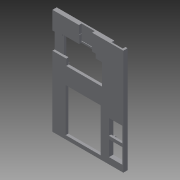
# Autodesk Inventor part: DisplayBottom2
Saved by Autodesk Inventor 2014 SP1 (Build 180222100, 222)
## iProperties
Created: 2014-03-24
Part Number: DisplayBottom2
Material: Generic
Document SubType Name: Modeling
Designer: patrigg
Density: 1 g/cm^3
Appearance: Default
Author: patrigg
Autodesk Inventor part; units mm, degrees
ref_plane "YZ Plane" through (0, 0, 0) normal (1, 0, 0) x (0, 1, 0)
ref_plane "XZ Plane" through (0, 0, 0) normal (0, 1, 0) x (-1, 0, 0)
ref_plane "XY Plane" through (0, 0, 0) normal (0, 0, 1) x (1, 0, 0)
sketch "Sketch2" plane through (0, 0, 0) normal (0, 1, 0) x (-1, 0, 0)
  line L0 (-33.5, -50) -> (33.5, -50)
  line L1 (33.5, -50) -> (33.5, 50)
  line L2 (33.5, 50) -> (-33.5, 50)
  line L3 (-33.5, 50) -> (-33.5, -50)
  line L4 (-33.5, -50) -> (33.5, 50) construction
  line L5 (33.5, -50) -> (-33.5, 50) construction
  point P0 (0, 0)
  dimension "d0" = 67
  dimension "d1" = 100
  constraints: 12 end point, 2 midpoint, 2 parallel, 1 horizontal, 1 perpendicular
  measures "d0" distance of L2.end L1.end
  measures "d1" distance of L1.end L0.end
extrude "Extrusion1" add sketch "Sketch2" along normal blind 4
sketch "Sketch3" plane through (0, 4, 0) normal (0, 1, 0) x (1, 0, 0)
  line L0 (33.5, 50) -> (-33.5, 50) projected
  line L1 (-23.5, -4.5) -> (14.5, -4.5)
  line L2 (14.5, -4.5) -> (14.5, 48)
  line L3 (14.5, 48) -> (-23.5, 48)
  line L4 (-23.5, 48) -> (-23.5, -4.5)
  line L5 (-23.5, -4.5) -> (14.5, 48) construction
  line L6 (14.5, -4.5) -> (-23.5, 48) construction
  line L7 (-33.5, 50) -> (-33.5, -50) projected
  point P0 (0, 0)
  point P1 (-4.5, 21.75)
  dimension "d4" = 38
  dimension "d5" = 52.5
  dimension "d6" = 2
  dimension "d111" = 10
  constraints: 12 end point, 2 midpoint, 2 parallel, 1 horizontal, 1 perpendicular
  measures "d4" distance of L3.end L2.end
  measures "d5" distance of L2.end L1.end
  measures "d6" distance between parallel lines of L0 L3
  measures "d111" distance between parallel lines of L4 L7
extrude "Extrusion2" cut sketch "Sketch3" against normal blind 1.5
sketch "Sketch4" plane through (0, 2.5, 0) normal (0, 1, 0) x (1, 0, 0)
  line L0 (14.5, -4.5) -> (-23.5, -4.5) projected
  line L1 (14.5, 48) -> (14.5, -4.5) projected
  line L2 (-23.5, 48) -> (14.5, 48) projected
  line L3 (-23.5, -4.5) -> (-23.5, 48) projected
  line L4 (-21, 46.5) -> (12, 46.5)
  line L5 (12, 46.5) -> (12, 5.5)
  line L6 (12, 5.5) -> (-21, 5.5)
  line L7 (-21, 5.5) -> (-21, 46.5)
  line L8 (-21, 46.5) -> (12, 5.5) construction
  line L9 (12, 46.5) -> (-21, 5.5) construction
  point P0 (0, 0)
  point P1 (-4.5, 26)
  dimension "d9" = 10
  dimension "d10" = 1.5
  dimension "d11" = 2.5
  dimension "d12" = 2.5
  constraints: 12 end point, 2 midpoint, 2 parallel, 1 horizontal, 1 perpendicular
  measures "d9" distance between parallel lines of L0 L6
  measures "d10" distance between parallel lines of L2 L4
  measures "d11" distance between parallel lines of L1 L5
  measures "d12" distance between parallel lines of L3 L7
extrude "Extrusion3" cut sketch "Sketch4" against normal blind 2.5 contours L4 L5 L6 L7
sketch "Sketch12" plane through (0, 4, 0) normal (0, 1, 0) x (1, 0, 0)
  line L0 (-24.5, -34.5) -> (13.5, -34.5)
  line L1 (13.5, -34.5) -> (13.5, -10.5)
  line L2 (13.5, -10.5) -> (-24.5, -10.5)
  line L3 (-24.5, -10.5) -> (-24.5, -34.5)
  line L4 (-24.5, -34.5) -> (13.5, -10.5) construction
  line L5 (13.5, -34.5) -> (-24.5, -10.5) construction
  line L6 (-23.5, -4.5) -> (-23.5, 48) projected
  line L7 (14.5, -4.5) -> (-23.5, -4.5) projected
  point P0 (0, 0)
  point P1 (-5.5, -22.5)
  point P2 (-5.5, -22.5)
  dimension "d58" = 38
  dimension "d59" = 24
  dimension "d112" = 1
  dimension "d154" = 6
  constraints: 12 end point, 3 midpoint, 2 parallel, 1 horizontal, 1 perpendicular
  measures "d58" distance of L2.end L1.end
  measures "d59" distance of L1.end L0.end
  measures "d112" distance between parallel lines of L3 L6
  measures "d154" distance between parallel lines of L7 L2
extrude "Extrusion10" cut sketch "Sketch12" against normal blind 4
sketch "Sketch18" plane through (13.5, 4, 10.5) normal (-1, 0, 0) x (0, 0, 1)
  line L0 (0, 0) -> (24, 0) projected
  line L1 (24, -4) -> (20, -4)
  line L2 (20, -4) -> (20, -1.8)
  line L3 (20, -1.8) -> (24, -1.8)
  line L4 (24, -1.8) -> (24, -4)
  point P0 (-10.5, -4)
  dimension "d88" = 4
  dimension "d89" = 1.8
  constraints: 8 end point, 2 parallel, 1 horizontal, 1 perpendicular
  measures "d88" distance of L2.end L3.end
  measures "d89" distance between parallel lines of L3 L0
extrude "Extrusion17" add sketch "Sketch18" along normal blind 6
sketch "Sketch20" plane through (-24.5, 4, 34.5) normal (1, 0, 0) x (0, 0, -1)
  line L0 (0, 0) -> (24, 0) projected
  line L1 (24, -4) -> (18, -4)
  line L2 (18, -4) -> (18, -1.8)
  line L3 (18, -1.8) -> (24, -1.8)
  line L4 (24, -1.8) -> (24, -4)
  point P0 (34.5, -4)
  dimension "d96" = 6
  dimension "d97" = 1.8
  constraints: 8 end point, 2 parallel, 1 horizontal, 1 perpendicular
  measures "d96" distance of L2.end L3.end
  measures "d97" distance between parallel lines of L3 L0
extrude "Extrusion19" add sketch "Sketch20" along normal blind 4
sketch "Sketch22" plane through (0, 0, 0) normal (0, -1, 0) x (1, 0, 0)
  line L0 (33.5, 50) -> (33.5, -50) projected
  line L1 (32.5, -44) -> (20, -44)
  line L2 (20, -44) -> (20, -12)
  line L3 (20, -12) -> (32.5, -12)
  line L4 (32.5, -12) -> (32.5, -44)
  line L5 (33.5, -50) -> (-33.5, -50) projected
  point P0 (0, 0)
  dimension "d102" = 1
  dimension "d103" = 12.5
  dimension "d110" = 32
  dimension "d155" = 6
  constraints: 8 end point, 2 parallel, 1 horizontal, 1 perpendicular
  measures "d102" distance between parallel lines of L4 L0
  measures "d103" distance between parallel lines of L2 L4
  measures "d110" distance between parallel lines of L3 L1
  measures "d155" distance between parallel lines of L5 L1
extrude "Extrusion21" cut sketch "Sketch22" against normal up to next
sketch "Sketch23" plane through (0, 4, 0) normal (0, 1, 0) x (1, 0, 0)
  line L0 (-24.5, -10.5) -> (13.5, -10.5) projected
  line L1 (14.5, 48) -> (14.5, -4.5) projected
  line L2 (14.5, -4.5) -> (-23.5, -4.5) projected
  line L3 (-23.5, -4.5) -> (-23.5, 48) projected
  line L4 (-21.5, -4.5) -> (-21.5, -10.5)
  line L5 (12.5, -4.5) -> (12.5, -10.5)
  point P0 (0, 0)
  dimension "d114" = 2
  dimension "d115" = 2
  constraints: 4 end point, 4 point on line, 2 perpendicular
  measures "d114" distance between parallel lines of L4 L3
  measures "d115" distance between parallel lines of L1 L5
extrude "Extrusion22" cut sketch "Sketch23" against normal up to surface (1.5 mm away)
sketch "Sketch24" plane through (32.5, 0, -44) normal (-1, 0, 0) x (0, 0, 1)
  line L0 (0, 0) -> (0, 4) projected
  line L1 (32, 0) -> (0, 0) projected
  line L2 (14.5, 0) -> (17.5, 0)
  line L3 (17.5, 0) -> (17.5, 2)
  line L4 (17.5, 2) -> (14.5, 2)
  line L5 (14.5, 2) -> (14.5, 0)
  line L6 (14.5, 0) -> (17.5, 2) construction
  line L7 (17.5, 0) -> (14.5, 2) construction
  point P0 (16, 1)
  dimension "d118" = 3
  dimension "d119" = 2
  dimension "d120" = 16
  constraints: 12 end point, 2 midpoint, 2 parallel, 1 collinear, 1 horizontal, 1 perpendicular
  measures "d118" distance of L4.end L3.end
  measures "d119" distance of L3.end L2.end
  measures "d120" distance from line of L0 point (16, 1)
extrude "Extrusion23" add sketch "Sketch24" along normal up to next
sketch "Sketch25" plane through (32.5, 2, -26.5) normal (0, 1, 0) x (1, 0, 0)
  line L0 (0, 0) -> (-12.5, 0) projected
  line L1 (0, 3) -> (-12.5, 3) projected
  line L2 (-7.75, 1) -> (-4.75, 1)
  line L3 (-4.75, 1) -> (-4.75, 3)
  line L4 (-4.75, 3) -> (-7.75, 3)
  line L5 (-7.75, 3) -> (-7.75, 1)
  line L6 (-7.75, 1) -> (-4.75, 3) construction
  line L7 (-4.75, 1) -> (-7.75, 3) construction
  point P0 (-32.5, -26.5)
  point P1 (-6.25, 2)
  point P2 (-6.25, 2)
  point P3 (-6.25, 0)
  dimension "d123" = 3
  dimension "d124" = 2
  constraints: 12 end point, 4 midpoint, 2 parallel, 1 collinear, 1 horizontal, 1 perpendicular, 1 vertical alignment
  measures "d123" distance of L4.end L3.end
  measures "d124" distance of L3.end L2.end
extrude "Extrusion24" cut sketch "Sketch25" against normal blind 0.5
fillet "Fillet6" radius 1 1 edges at (26.25, 1.5, -29.5)
sketch "Sketch26" plane through (32.5, 2, -26.5) normal (0, 1, 0) x (1, 0, 0)
  line L0 (0, 0) -> (-12.5, 0) projected
  line L1 (0, 3) -> (0, 0) projected
  circle A0 centre (-10.375, 1.5) radius 1.25
  circle A1 centre (-2.125, 1.5) radius 1.25
  point P0 (-32.5, -26.5)
  point P1 (-6.25, 1.5)
  point P2 (0, 1.5)
  point P3 (-6.25, 0)
  dimension "d128" = 2.5
  dimension "d129" = 2.5
  dimension "d130" = 4.125
  dimension "d131" = 8.25
  constraints: 3 horizontal alignment, 2 centre point, 2 midpoint, 1 vertical alignment
  measures "d128" diameter of A0
  measures "d129" diameter of A1
  measures "d130" distance of point (-6.25, 1.5) A0.centre
  measures "d131" distance of A1.centre A0.centre
extrude "Extrusion25" add sketch "Sketch26" along normal blind 2
chamfer "Chamfer3" distance 0.5 angle 45 2 edges at (29.125, 4, -28) (20.875, 4, -28)
sketch "Sketch27" plane through (0, 4, 0) normal (0, 1, 0) x (1, 0, 0)
  line L0 (-33.5, -50) -> (33.5, -50) projected
  line L1 (32.5, 12) -> (20, 12) projected
  line L2 (20, 44) -> (32.5, 44) projected
  line L3 (21, -50) -> (31.5, -50)
  line L4 (31.5, -50) -> (31.5, -32)
  line L5 (31.5, -32) -> (21, -32)
  line L6 (21, -32) -> (21, -50)
  line L7 (21, -50) -> (31.5, -32) construction
  line L8 (31.5, -50) -> (21, -32) construction
  line L9 (20, 12) -> (20, 44) projected
  line L10 (21, -42) -> (21.25, -42)
  line L11 (21.25, -42) -> (21.25, -32)
  line L12 (31.5, -42) -> (31.25, -42)
  line L13 (31.25, -42) -> (31.25, -32)
  point P0 (0, 0)
  point P1 (26.25, 44)
  point P2 (26.25, -41)
  point P3 (26.25, -41)
  point P4 (26.25, 12)
  dimension "d138" = 10.5
  dimension "d139" = 18
  dimension "d148" = 0.25
  dimension "d149" = 0.25
  dimension "d150" = 8
  constraints: 20 end point, 5 midpoint, 5 perpendicular, 4 point on line, 2 collinear, 2 parallel, 1 horizontal, 1 vertical alignment
  measures "d138" distance of L5.end L4.end
  measures "d139" distance of L4.end L3.end
  measures "d148" distance between parallel lines of L11 L6
  measures "d149" distance between parallel lines of L4 L13
  measures "d150" distance from line of L0 L10.end
extrude "Extrusion26" cut sketch "Sketch27" against normal blind 2.5 contours L6 L10 L11 L5 L13 L12 L4 L0
sketch "Sketch28" plane through (0, 4, 0) normal (0, 1, 0) x (1, 0, 0)
  line L0 (32.5, 12) -> (20, 12) projected
  line L1 (21.25, -32) -> (31.25, -32) projected
  line L2 (23.75, 12) -> (28.75, 12)
  line L3 (28.75, 12) -> (28.75, -32)
  line L4 (28.75, -32) -> (23.75, -32)
  line L5 (23.75, -32) -> (23.75, 12)
  line L6 (23.75, 12) -> (28.75, -32) construction
  line L7 (28.75, 12) -> (23.75, -32) construction
  point P0 (21, -27)
  point P1 (31.5, -27)
  point P2 (0, 0)
  point P3 (26.25, -10)
  point P4 (26.25, -10)
  point P5 (26.25, 12)
  dimension "d142" = 5
  constraints: 12 end point, 4 midpoint, 2 horizontal, 2 parallel, 1 collinear, 1 perpendicular, 1 vertical alignment, 1 other
  measures "d142" distance between parallel lines of L3 L5
extrude "Extrusion27" cut sketch "Sketch28" against normal blind 1
chamfer "Chamfer4" distance 1 angle 45 2 edges at (26.25, 3, 32) (26.25, 3, -12)
sketch "Sketch29" plane through (0, 0, 0) normal (0, -1, 0) x (1, 0, 0)
  line L0 (-24.5, 16.5) -> (-24.5, 34.5) projected
  line L1 (-24.5, 34.5) -> (7.5, 34.5) projected
  line L2 (-33.5, -50) -> (-33.5, 50) projected
  line L3 (-33.5, 50) -> (33.5, 50) projected
  line L4 (-24.5, 16.5) -> (-33.5, 16.5)
  line L5 (-24.5, 33) -> (-33.5, 33)
  point P0 (0, 0)
  dimension "d151" = 1.5
  constraints: 4 end point, 3 point on line, 1 parallel, 1 perpendicular
  measures "d151" distance between parallel lines of L1 L5
extrude "Extrusion28" cut sketch "Sketch29" against normal blind 2
sketch "Sketch30" plane through (0, 0, 0) normal (0, -1, 0) x (1, 0, 0)
  line L0 (-33.5, 50) -> (33.5, 50) projected
  line L1 (-8.5, 42) -> (4, 42)
  line L2 (4, 42) -> (4, 50)
  line L3 (4, 50) -> (-8.5, 50)
  line L4 (-8.5, 50) -> (-8.5, 42)
  line L5 (-8.5, 42) -> (4, 50) construction
  line L6 (4, 42) -> (-8.5, 50) construction
  line L7 (3.75, 36) -> (-8.25, 36)
  line L8 (-8.25, 36) -> (-8.25, 42)
  line L9 (-8.25, 42) -> (3.75, 42)
  line L10 (3.75, 42) -> (3.75, 36)
  line L11 (3.75, 36) -> (-8.25, 42) construction
  line L12 (-8.25, 36) -> (3.75, 42) construction
  point P0 (-24.5, 34.5)
  point P1 (0, 0)
  point P2 (-2.25, 46)
  point P3 (-2.25, 39)
  point P4 (-2.25, 39)
  point P5 (-2.25, 46)
  dimension "d156" = 12.5
  dimension "d157" = 8
  dimension "d158" = 16
  dimension "d162" = 12
  dimension "d164" = 6
  constraints: 24 end point, 6 midpoint, 4 parallel, 2 horizontal, 2 perpendicular, 1 collinear, 1 point on line, 1 vertical alignment
  measures "d156" distance of L3.end L2.end
  measures "d157" distance of L2.end L1.end
  measures "d158" distance from line of L4 point (-24.5, 34.5)
  measures "d162" distance between parallel lines of L8 L10
  measures "d164" distance between parallel lines of L9 L7
extrude "Extrusion29" cut sketch "Sketch30" against normal blind 2.5
sketch "Sketch31" plane through (0, 0, 0) normal (0, -1, 0) x (1, 0, 0)
  line L0 (-24.5, 34.5) -> (7.5, 34.5) projected
  line L1 (3.75, 42) -> (3.75, 36) projected
  line L2 (3.75, 36) -> (-8.25, 36) projected
  line L3 (-8.25, 36) -> (-8.25, 42) projected
  line L4 (20, -44) -> (20, -29.5) projected
  line L5 (3.75, 34.5) -> (3.75, 36)
  line L6 (-8.25, 34.5) -> (-8.25, 36)
  point P0 (0, 0)
  constraints: 4 end point, 4 point on line, 2 collinear, 1 parallel, 1 perpendicular
extrude "Extrusion30" cut sketch "Sketch31" against normal blind 2
body "Solid1"
